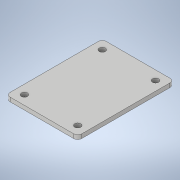
# Autodesk Inventor part: Tampa
Saved by Autodesk Inventor 2021 (Build 250183000, 183)
## iProperties
Created: 2021-05-27
Part Number: Tampa
Material: Generic
Document SubType Name: Modeling
Designer: hoope
Density: 1 g/cm^3
Appearance: Default
Author: hoope
Autodesk Inventor part; units mm, degrees
ref_plane "YZ Plane" through (0, 0, 0) normal (1, 0, 0) x (0, 1, 0)
ref_plane "XZ Plane" through (0, 0, 0) normal (0, 1, 0) x (-1, 0, 0)
ref_plane "XY Plane" through (0, 0, 0) normal (0, 0, 1) x (1, 0, 0)
sketch "Esboço1" plane through (0, 0, 0) normal (0, 1, 0) x (-1, 0, 0)
  line L0 (0, 0) -> (35, 0)
  line L1 (35, 0) -> (35, -47)
  line L2 (35, -47) -> (0, -47)
  line L3 (0, -47) -> (0, 0)
  dimension "d0" = 35
  dimension "d1" = 47
  constraints: 8 end point, 2 parallel, 1 horizontal, 1 perpendicular
  measures "d0" distance of L1.end L2.end
  measures "d1" distance of L0.end L1.end
extrude "Extrusão1" add sketch "Esboço1" along normal blind 2
fillet "Arredondamento1" radius 2 4 edges at (0, 1, 0) (0, 1, -47) (-35, 1, 0) (-35, 1, -47)
sketch "Esboço5" plane through (0, 2, 0) normal (0, 1, 0) x (1, 0, 0)
  circle A0 centre (-4.5, 42.5) radius 1.505
  line L0 (-2, 47) -> (-33, 47) projected
  line L1 (0, 2) -> (0, 45) projected
  circle A1 centre (-30.5, 42.5) radius 1.505
  circle A2 centre (-4.5, 4.5) radius 1.505
  circle A3 centre (-30.5, 4.5) radius 1.505
  point P0 (0, 0)
  dimension "d26" = 3.01
  dimension "d27" = 4.5
  dimension "d28" = 4.5
  dimension "d31" = 26
  dimension "d34" = 38
  constraints: 4 centre point, 1 horizontal, 1 vertical, 6 other
  measures "d26" diameter of A0
  measures "d27" distance from line of L0 A0.centre
  measures "d28" distance from line of L1 A0.centre
  measures "d31" distance of A0.centre A1.centre
  measures "d34" distance of A0.centre A2.centre
extrude "Extrusão4" cut sketch "Esboço5" against normal blind 4.5
equation "\"d37\" = d28"
